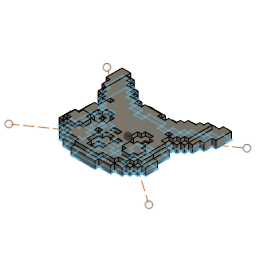
pikatchu v1 (Autodesk Fusion 360 design; units mm, degrees)
Autodesk Fusion 360 part; units mm, degrees
note: some values were not read from the file. Chosen so that the rebuilt part matches the saved one: which bodies a step acts on.
sketch "pikatchu" plane through (0, 0, 0) normal (0, 1, 0) x (1, 0, 0)
  line L0 (5, -3.5) -> (-5, 3.5) construction
  line L1 (-5, -3.5) -> (5, 3.5) construction
  line L2 (-3.9, 3.5) -> (-3.3, 3.5)
  line L3 (-3.3, 3.5) -> (-3.3, 3.2)
  line L4 (-3.3, 3.2) -> (-2.75, 3.2)
  line L5 (-2.75, 3.2) -> (-2.75, 2.9237)
  line L6 (-2.75, 2.9237) -> (-2.4765, 2.9237)
  line L7 (-2.4765, 2.9237) -> (-2.4765, 2.65)
  line L8 (-2.4765, 2.65) -> (-1.92, 2.65)
  line L9 (-1.92, 2.65) -> (-1.92, 2.365)
  line L10 (-1.92, 2.365) -> (-1.65, 2.365)
  line L11 (-1.65, 2.365) -> (-1.65, 2.1)
  line L12 (-1.65, 2.1) -> (-1.1, 2.1)
  line L13 (-1.1, 2.1) -> (-1.1, 1.8)
  line L14 (-1.1, 1.8) -> (-0.5805, 1.8)
  line L15 (-0.5805, 1.8) -> (-0.5805, 2.1)
  line L16 (-0.5805, 2.1) -> (0.5819, 2.1)
  line L17 (0.5819, 2.1) -> (0.5819, 1.8)
  line L18 (0.5819, 1.8) -> (1.1, 1.8)
  line L19 (1.1, 1.8) -> (1.1, 2.1)
  line L20 (1.1, 2.1) -> (1.65, 2.1)
  line L21 (1.65, 2.1) -> (1.65, 2.3687)
  line L22 (1.65, 2.3687) -> (1.9285, 2.3687)
  line L23 (1.9285, 2.3687) -> (1.9285, 2.65)
  line L24 (1.9285, 2.65) -> (2.4811, 2.65)
  line L25 (2.4811, 2.65) -> (2.4811, 2.9274)
  line L26 (2.4811, 2.9274) -> (2.7659, 2.9274)
  line L27 (2.7659, 2.9274) -> (2.7659, 3.2)
  line L28 (2.7659, 3.2) -> (3.3216, 3.2)
  line L29 (3.3216, 3.2) -> (3.3216, 3.4831)
  line L30 (3.3216, 3.4831) -> (3.9144, 3.4831)
  line L31 (3.9144, 3.4831) -> (3.9144, 2.3719)
  line L32 (3.9144, 2.3719) -> (3.6327, 2.3719)
  line L33 (3.6327, 2.3719) -> (3.6327, 1.8)
  line L34 (3.6327, 1.8) -> (3.3481, 1.8)
  line L35 (3.3481, 1.8) -> (3.3481, 1.2593)
  line L36 (3.3481, 1.2593) -> (3.0744, 1.2593)
  line L37 (3.0744, 1.2593) -> (3.0744, 0.9693)
  line L38 (3.0744, 0.9693) -> (2.8, 0.9693)
  line L39 (2.8, 0.9693) -> (2.8, 0.7)
  line L40 (2.8, 0.7) -> (2.523, 0.7)
  line L41 (2.523, 0.7) -> (2.523, 0.15)
  line L42 (2.523, 0.15) -> (2.8, 0.15)
  line L43 (2.8, 0.15) -> (2.8, -0.97)
  line L44 (2.8, -0.97) -> (3.08, -0.97)
  line L45 (3.08, -0.97) -> (3.08, -1.81)
  line L46 (3.08, -1.81) -> (2.8, -1.81)
  line L47 (2.8, -1.81) -> (2.8, -2.1)
  line L48 (2.8, -2.1) -> (2.52, -2.1)
  line L49 (2.52, -2.1) -> (2.52, -2.37)
  line L50 (2.52, -2.37) -> (2.24, -2.37)
  line L51 (2.24, -2.37) -> (2.24, -2.65)
  line L52 (2.24, -2.65) -> (1.69, -2.65)
  line L53 (1.69, -2.65) -> (1.69, -2.9293)
  line L54 (1.69, -2.9293) -> (0.85, -2.9293)
  line L55 (0.85, -2.9293) -> (0.85, -3.2)
  line L56 (0.85, -3.2) -> (-0.8573, -3.2)
  line L57 (-0.8573, -3.2) -> (-0.8573, -2.9293)
  line L58 (-0.8573, -2.9293) -> (-1.7, -2.9293)
  line L59 (-1.7, -2.9293) -> (-1.7, -2.65)
  line L60 (-1.7, -2.65) -> (-2.2349, -2.65)
  line L61 (-2.2349, -2.65) -> (-2.2349, -2.3726)
  line L62 (-2.2349, -2.3726) -> (-2.5262, -2.3726)
  line L63 (-2.5262, -2.3726) -> (-2.5262, -2.1)
  line L64 (-2.5262, -2.1) -> (-2.8043, -2.1)
  line L65 (-2.8043, -2.1) -> (-2.8043, -1.82)
  line L66 (-2.8043, -1.82) -> (-3.09, -1.82)
  line L67 (-3.09, -1.82) -> (-3.09, -0.9667)
  line L68 (-3.09, -0.9667) -> (-2.8043, -0.9667)
  line L69 (-2.8043, -0.9667) -> (-2.8043, 0.1465)
  line L70 (-2.8043, 0.1465) -> (-2.5283, 0.1465)
  line L71 (-2.5283, 0.1465) -> (-2.5283, 0.7)
  line L72 (-2.5283, 0.7) -> (-2.8, 0.7)
  line L73 (-2.8, 0.7) -> (-2.8, 0.966)
  line L74 (-2.8, 0.966) -> (-3.09, 0.966)
  line L75 (-3.09, 0.966) -> (-3.09, 1.24)
  line L76 (-3.09, 1.24) -> (-3.37, 1.24)
  line L77 (-3.37, 1.24) -> (-3.37, 1.8)
  line L78 (-3.37, 1.8) -> (-3.65, 1.8)
  line L79 (-3.65, 1.8) -> (-3.65, 2.36)
  line L80 (-3.65, 2.36) -> (-3.92, 2.36)
  line L81 (-3.92, 2.36) -> (-3.92, 3.5)
  line L82 (-3.92, 3.5) -> (-3.9, 3.5)
  line L83 (-2.75, 2.9237) -> (-3.05, 2.9237)
  line L84 (-3.05, 2.9237) -> (-3.05, 1.24)
  line L85 (-3.05, 1.24) -> (-2.8, 1.24)
  line L86 (-2.8, 1.24) -> (-2.8, 0.966)
  line L87 (-2.5283, 0.966) -> (-2.5283, 0.7)
  line L88 (-2.8, 0.966) -> (-2.5283, 0.966)
  line L89 (-2.5283, 0.7) -> (-2.2385, 0.7)
  line L90 (-2.2385, 0.7) -> (-2.2385, 0.9761)
  line L91 (-2.2385, 0.9761) -> (-1.95, 0.9761)
  line L92 (-1.95, 0.9761) -> (-1.95, 0.7)
  line L93 (-1.95, 0.7) -> (-2.2385, 0.7)
  line L94 (-2.2385, 0.1465) -> (-2.5283, 0.1465)
  line L95 (-2.2385, 0.7) -> (-2.2385, 0.1465)
  line L96 (-2.5283, 0.1465) -> (-2.5283, -0.9667)
  line L97 (-2.5283, -0.9667) -> (-2.8043, -0.9667)
  line L98 (-2.8043, -0.9667) -> (-2.8043, -1.82)
  line L99 (-2.8043, -1.82) -> (-2.5262, -1.82)
  line L100 (-2.5262, -1.82) -> (-2.5262, -1.2565)
  line L101 (-2.5262, -1.2565) -> (-2.2296, -1.2565)
  line L102 (-2.2296, -1.2565) -> (-2.2296, -0.9685)
  line L103 (-2.2296, -0.9685) -> (-1.7, -0.9685)
  line L104 (-1.7, -0.9685) -> (-1.7, -1.2565)
  line L105 (-1.7, -1.2565) -> (-1.4, -1.2565)
  line L106 (-1.4, -1.2565) -> (-1.4, -1.8)
  line L107 (-1.4, -1.8) -> (-1.6867, -1.8)
  line L108 (-1.6867, -1.8) -> (-1.6867, -2.1)
  line L109 (-1.6867, -2.1) -> (-2.2349, -2.1)
  line L110 (-2.2349, -2.1) -> (-2.2349, -1.82)
  line L111 (-2.2349, -1.82) -> (-2.5262, -1.82)
  line L112 (-2.5262, -1.82) -> (-2.5262, -2.1)
  line L113 (-2.5262, -2.1) -> (-2.2349, -2.1)
  line L114 (-2.2349, -2.1) -> (-2.2349, -2.3726)
  line L115 (-2.2349, -2.3726) -> (-1.7, -2.3726)
  line L116 (-1.7, -2.3726) -> (-1.7, -2.65)
  line L117 (-1.7, -2.65) -> (-0.8573, -2.65)
  line L118 (-0.8573, -2.65) -> (-0.8573, -2.9293)
  line L119 (-0.8573, -2.9293) -> (0.85, -2.9293)
  line L120 (0.85, -2.9293) -> (0.85, -2.65)
  line L121 (0.85, -2.65) -> (1.69, -2.65)
  line L122 (1.69, -2.65) -> (1.69, -2.37)
  line L123 (1.69, -2.37) -> (2.24, -2.37)
  line L124 (2.24, -2.37) -> (2.24, -2.1)
  line L125 (2.24, -2.1) -> (2.52, -2.1)
  line L126 (2.52, -2.1) -> (2.52, -1.81)
  line L127 (2.52, -1.81) -> (2.8, -1.81)
  line L128 (2.8, -0.97) -> (2.8, -1.81)
  line L129 (2.8, -0.97) -> (2.523, -0.97)
  line L130 (2.523, -0.97) -> (2.523, 0.15)
  line L131 (2.523, 0.15) -> (2.2342, 0.15)
  line L132 (2.2342, 0.15) -> (2.2342, 0.7)
  line L133 (2.2342, 0.7) -> (2.523, 0.7)
  line L134 (2.523, 0.7) -> (2.523, 0.9693)
  line L135 (2.523, 0.9693) -> (2.8, 0.9693)
  line L136 (2.2342, 0.7) -> (1.95, 0.7)
  line L137 (1.95, 0.7) -> (1.95, 0.9755)
  line L138 (1.95, 0.9755) -> (2.2342, 0.9755)
  line L139 (2.2342, 0.9755) -> (2.2342, 0.7)
  line L140 (2.8, 0.9693) -> (2.8, 1.2593)
  line L141 (2.8, 1.2593) -> (3.0744, 1.2593)
  line L142 (3.0744, 1.2593) -> (3.0744, 2.9274)
  line L143 (3.0744, 2.9274) -> (2.7659, 2.9274)
  line L144 (2.7659, 2.9274) -> (2.7659, 2.65)
  line L145 (2.7659, 2.65) -> (2.4811, 2.65)
  line L146 (2.4811, 2.65) -> (2.4811, 2.3687)
  line L147 (2.4811, 2.3687) -> (1.9285, 2.3687)
  line L148 (1.9285, 2.3687) -> (1.9285, 2.1)
  line L149 (1.9285, 2.1) -> (1.65, 2.1)
  line L150 (1.65, 2.1) -> (1.65, 1.8)
  line L151 (1.65, 1.8) -> (1.1, 1.8)
  line L152 (1.1, 1.8) -> (1.1, 1.5472)
  line L153 (1.1, 1.5472) -> (0.5819, 1.5472)
  line L154 (0.5819, 1.5472) -> (0.5819, 1.8)
  line L155 (0.5819, 1.8) -> (-0.5805, 1.8)
  line L156 (-0.5805, 1.8) -> (-0.5805, 1.55)
  line L157 (-0.5805, 1.55) -> (-1.1, 1.55)
  line L158 (-1.1, 1.55) -> (-1.1, 1.8)
  line L159 (-1.65, 2.1) -> (-1.65, 1.8)
  line L160 (-1.65, 1.8) -> (-1.1, 1.8)
  line L161 (-1.92, 2.365) -> (-1.92, 2.1)
  line L162 (-1.92, 2.1) -> (-1.65, 2.1)
  line L163 (-1.92, 2.365) -> (-2.4765, 2.365)
  line L164 (-2.4765, 2.365) -> (-2.4765, 2.65)
  line L165 (-2.75, 2.9237) -> (-2.75, 2.65)
  line L166 (-2.75, 2.65) -> (-2.4765, 2.65)
  line L167 (0.27, -2.35) -> (-0.27, -2.35)
  line L168 (-0.27, -2.35) -> (-0.27, -1.82)
  line L169 (-0.27, -1.82) -> (0.27, -1.82)
  line L170 (0.27, -1.82) -> (0.27, -2.35)
  line L171 (-0.27, -2.35) -> (-0.27, -2.65)
  line L172 (-0.27, -2.65) -> (0.27, -2.65)
  line L173 (0.27, -2.65) -> (0.27, -2.35)
  line L174 (0.27, -2.35) -> (0.5454, -2.35)
  line L175 (0.5454, -2.35) -> (0.5454, -1.5281)
  line L176 (0.5454, -1.5281) -> (0.8298, -1.5281)
  line L177 (0.8298, -1.5281) -> (0.8298, -1.2462)
  line L178 (0.8298, -1.2462) -> (0.5454, -1.2462)
  line L179 (0.5454, -1.2462) -> (0.5454, -1.5281)
  line L180 (0.2686, -1.5281) -> (0.2686, -1.2462)
  line L181 (0.2686, -1.2462) -> (-0.2864, -1.2462)
  line L182 (-0.2864, -1.2462) -> (-0.2864, -1.5281)
  line L183 (-0.2864, -1.5281) -> (-0.56, -1.5281)
  line L184 (-0.56, -1.5281) -> (-0.56, -1.2462)
  line L185 (-0.56, -1.2462) -> (-0.84, -1.2462)
  line L186 (-0.84, -1.2462) -> (-0.84, -1.5281)
  line L187 (-0.84, -1.5281) -> (-0.56, -1.5281)
  line L188 (-0.56, -1.5281) -> (-0.56, -2.35)
  line L189 (-0.56, -2.35) -> (-0.27, -2.35)
  line L190 (0.2686, -1.5281) -> (0.5454, -1.5281)
  line L191 (0.2673, -0.6984) -> (0.2673, -0.9849)
  line L192 (0.2673, -0.9849) -> (-0.2867, -0.9849)
  line L193 (-0.2867, -0.9849) -> (-0.2867, -0.6984)
  line L194 (-0.2867, -0.6984) -> (0.2673, -0.6984)
  line L195 (1.4, -1.2567) -> (1.4, -1.8)
  line L196 (1.4, -1.8) -> (1.6685, -1.8)
  line L197 (1.6685, -1.8) -> (1.6685, -2.1)
  line L198 (1.6685, -2.1) -> (2.24, -2.1)
  line L199 (2.24, -2.1) -> (2.24, -1.81)
  line L200 (2.24, -1.81) -> (2.52, -1.81)
  line L201 (2.52, -1.81) -> (2.52, -1.26)
  line L202 (2.52, -1.26) -> (2.22, -1.26)
  line L203 (2.22, -1.26) -> (2.22, -0.98)
  line L204 (2.22, -0.98) -> (1.66, -0.98)
  line L205 (1.66, -0.98) -> (1.66, -1.2567)
  line L206 (1.66, -1.2567) -> (1.4, -1.2567)
  line L207 (-1.7, -0.9685) -> (-1.1247, -0.9685)
  line L208 (-1.1247, -0.9685) -> (-1.1247, -0.69)
  line L209 (-1.1247, -0.69) -> (-0.84, -0.69)
  line L210 (-0.84, -0.69) -> (-0.84, -0.14)
  line L211 (-0.84, -0.14) -> (-1.1247, -0.14)
  line L212 (-1.1247, -0.14) -> (-1.1247, 0.14)
  line L213 (-1.1247, 0.14) -> (-1.68, 0.14)
  line L214 (-1.68, 0.14) -> (-1.68, -0.14)
  line L215 (-1.68, -0.14) -> (-1.96, -0.14)
  line L216 (-1.96, -0.14) -> (-1.96, -0.69)
  line L217 (-1.96, -0.69) -> (-1.7, -0.69)
  line L218 (-1.7, -0.69) -> (-1.7, -0.9685)
  line L219 (-1.68, -0.14) -> (-1.4, -0.14)
  line L220 (-1.4, -0.14) -> (-1.4, -0.4152)
  line L221 (-1.4, -0.4152) -> (-1.68, -0.4152)
  line L222 (-1.68, -0.4152) -> (-1.68, -0.14)
  line L223 (1.66, -0.98) -> (1.66, -0.7)
  line L224 (1.66, -0.7) -> (1.94, -0.7)
  line L225 (1.94, -0.7) -> (1.94, -0.14)
  line L226 (1.94, -0.14) -> (1.67, -0.14)
  line L227 (1.67, -0.14) -> (1.67, 0.14)
  line L228 (1.67, 0.14) -> (1.1, 0.14)
  line L229 (1.1, 0.14) -> (1.1, -0.14)
  line L230 (1.1, -0.14) -> (0.83, -0.14)
  line L231 (0.83, -0.14) -> (0.83, -0.7)
  line L232 (0.83, -0.7) -> (1.1, -0.7)
  line L233 (1.1, -0.7) -> (1.1, -0.98)
  line L234 (1.1, -0.98) -> (1.66, -0.98)
  line L235 (1.67, -0.14) -> (1.4, -0.14)
  line L236 (1.4, -0.14) -> (1.4, -0.41)
  line L237 (1.4, -0.41) -> (1.67, -0.41)
  line L238 (1.67, -0.41) -> (1.67, -0.14)
  dimension "d1" = 7
  dimension "d2" = 10
  dimension "d13" = 0.54
  constraint coincident L0 origin
  constraint coincident L1 origin
  constraint horizontal L2
  constraint perpendicular L2 L3
  constraint perpendicular L3 L4
  constraint perpendicular L4 L5
  constraint perpendicular L5 L6
  constraint perpendicular L6 L7
  constraint perpendicular L5 L8
  constraint perpendicular L8 L9
  constraint perpendicular L9 L10
  constraint perpendicular L10 L11
  constraint perpendicular L11 L12
  constraint perpendicular L10 L13
  constraint perpendicular L13 L14
  constraint perpendicular L10 L15
  constraint perpendicular L15 L16
  constraint perpendicular L16 L17
  constraint perpendicular L17 L18
  constraint perpendicular L18 L19
  constraint perpendicular L19 L20
  constraint perpendicular L18 L21
  constraint perpendicular L19 L22
  constraint perpendicular L18 L23
  constraint perpendicular L19 L24
  constraint perpendicular L18 L25
  constraint perpendicular L25 L26
  constraint perpendicular L26 L27
  constraint perpendicular L27 L28
  constraint perpendicular L26 L29
  constraint perpendicular L27 L30
  constraint perpendicular L26 L31
  constraint perpendicular L31 L32
  constraint perpendicular L26 L33
  constraint perpendicular L33 L34
  constraint perpendicular L34 L35
  constraint perpendicular L35 L36
  constraint perpendicular L36 L37
  constraint perpendicular L37 L38
  constraint perpendicular L38 L39
  constraint perpendicular L39 L40
  constraint perpendicular L38 L41
  constraint perpendicular L39 L42
  constraint perpendicular L42 L43
  constraint perpendicular L43 L44
  constraint perpendicular L42 L45
  constraint perpendicular L45 L46
  constraint perpendicular L46 L47
  constraint perpendicular L47 L48
  constraint perpendicular L46 L49
  constraint perpendicular L49 L50
  constraint perpendicular L50 L51
  constraint perpendicular L49 L52
  constraint perpendicular L52 L53
  constraint perpendicular L49 L54
  constraint perpendicular L54 L55
  constraint perpendicular L55 L56
  constraint perpendicular L56 L57
  constraint perpendicular L55 L58
  constraint perpendicular L58 L59
  constraint perpendicular L59 L60
  constraint perpendicular L60 L61
  constraint perpendicular L59 L62
  constraint perpendicular L62 L63
  constraint perpendicular L63 L64
  constraint perpendicular L64 L65
  constraint perpendicular L63 L66
  constraint perpendicular L64 L67
  constraint perpendicular L67 L68
  constraint perpendicular L68 L69
  constraint perpendicular L69 L70
  constraint perpendicular L70 L71
  constraint perpendicular L71 L72
  constraint perpendicular L70 L73
  constraint perpendicular L73 L74
  constraint perpendicular L74 L75
  constraint perpendicular L73 L76
  constraint perpendicular L74 L77
  constraint perpendicular L73 L78
  constraint perpendicular L78 L79
  constraint perpendicular L73 L80
  constraint perpendicular L80 L81
  constraint perpendicular L81 L82
  constraint perpendicular L5 L83
  constraint perpendicular L83 L84
  constraint perpendicular L84 L85
  constraint parallel L74 L88
  constraint perpendicular L87 L88
  constraint perpendicular L87 L89
  constraint perpendicular L89 L90
  constraint perpendicular L90 L91
  constraint perpendicular L91 L92
  constraint perpendicular L90 L93
  constraint parallel L92 L95
  constraint perpendicular L94 L95
  constraint perpendicular L94 L96
  constraint perpendicular L96 L97
  constraint perpendicular L66 L98
  constraint perpendicular L98 L99
  constraint perpendicular L66 L100
  constraint perpendicular L100 L101
  constraint perpendicular L101 L102
  constraint perpendicular L102 L103
  constraint perpendicular L101 L104
  constraint perpendicular L104 L105
  constraint perpendicular L105 L106
  constraint perpendicular L106 L107
  constraint perpendicular L106 L109
  constraint perpendicular L109 L110
  constraint perpendicular L110 L111
  constraint perpendicular L107 L108
  constraint perpendicular L64 L112
  constraint perpendicular L62 L114
  constraint perpendicular L61 L115
  constraint perpendicular L115 L116
  constraint perpendicular L59 L117
  constraint perpendicular L117 L118
  constraint perpendicular L55 L119
  constraint perpendicular L54 L120
  constraint perpendicular L120 L121
  constraint perpendicular L121 L122
  constraint perpendicular L122 L123
  constraint perpendicular L50 L124
  constraint perpendicular L124 L125
  constraint perpendicular L48 L126
  constraint perpendicular L126 L127
  constraint perpendicular L44 L128
  constraint perpendicular L128 L129
  constraint perpendicular L129 L130
  constraint perpendicular L130 L131
  constraint perpendicular L131 L132
  constraint perpendicular L41 L133
  constraint perpendicular L133 L134
  constraint perpendicular L134 L135
  constraint perpendicular L132 L136
  constraint perpendicular L136 L137
  constraint perpendicular L132 L138
  constraint perpendicular L133 L139
  constraint perpendicular L38 L140
  constraint perpendicular L140 L141
  constraint perpendicular L36 L142
  constraint perpendicular L142 L143
  constraint perpendicular L143 L144
  constraint perpendicular L27 L145
  constraint perpendicular L145 L146
  constraint perpendicular L146 L147
  constraint perpendicular L22 L148
  constraint perpendicular L149 L150
  constraint parallel L151 L153
  constraint perpendicular L148 L149
  constraint perpendicular L150 L151
  constraint perpendicular L152 L153
  constraint perpendicular L18 L154
  constraint perpendicular L15 L155
  constraint perpendicular L14 L156
  constraint perpendicular L15 L157
  constraint perpendicular L14 L158
  constraint perpendicular L12 L159
  constraint perpendicular L158 L160
  constraint perpendicular L10 L161
  constraint perpendicular L161 L163
  constraint perpendicular L163 L164
  constraint perpendicular L164 L166
  constraint perpendicular L165 L166
  constraint horizontal L167
  constraint perpendicular L167 L168
  constraint perpendicular L168 L169
  constraint perpendicular L167 L170
  constraint perpendicular L167 L171
  constraint perpendicular L171 L172
  constraint perpendicular L172 L173
  constraint perpendicular L173 L174
  constraint perpendicular L174 L175
  constraint perpendicular L173 L176
  constraint perpendicular L176 L177
  constraint perpendicular L173 L178
  constraint perpendicular L178 L179
  constraint perpendicular L178 L180
  constraint perpendicular L180 L181
  constraint perpendicular L178 L182
  constraint perpendicular L180 L183
  constraint perpendicular L183 L184
  constraint perpendicular L184 L185
  constraint perpendicular L185 L186
  constraint perpendicular L184 L187
  constraint perpendicular L187 L188
  constraint perpendicular L188 L189
  constraint perpendicular L179 L190
  constraint vertical L191
  constraint perpendicular L191 L192
  constraint perpendicular L192 L193
  constraint perpendicular L191 L194
  constraint perpendicular L194 L195
  constraint perpendicular L195 L196
  constraint perpendicular L194 L197
  constraint perpendicular L197 L198
  constraint perpendicular L125 L199
  constraint perpendicular L199 L200
  constraint perpendicular L127 L201
  constraint perpendicular L126 L202
  constraint perpendicular L126 L204
  constraint perpendicular L202 L203
  constraint perpendicular L204 L205
  constraint perpendicular L205 L206
  constraint perpendicular L104 L207
  constraint perpendicular L207 L208
  constraint perpendicular L208 L209
  constraint perpendicular L207 L210
  constraint perpendicular L210 L211
  constraint perpendicular L211 L212
  constraint perpendicular L212 L213
  constraint perpendicular L211 L214
  constraint perpendicular L214 L215
  constraint perpendicular L211 L216
  constraint perpendicular L214 L217
  constraint perpendicular L217 L218
  constraint perpendicular L214 L219
  constraint perpendicular L219 L220
  constraint perpendicular L214 L221
  constraint perpendicular L215 L222
  constraint perpendicular L204 L223
  constraint perpendicular L205 L224
  constraint perpendicular L204 L225
  constraint perpendicular L205 L226
  constraint perpendicular L226 L227
  constraint perpendicular L205 L228
  constraint perpendicular L226 L229
  constraint perpendicular L205 L230
  constraint perpendicular L226 L231
  constraint perpendicular L231 L232
  constraint perpendicular L226 L233
  constraint perpendicular L233 L234
  constraint perpendicular L227 L235
  constraint perpendicular L226 L236
  constraint perpendicular L227 L237
  constraint perpendicular L235 L238
  measures "d1" distance of L1.start L0.end
  measures "d2" distance of L0.end L1.end
  measures "d13" distance of L168 L170
extrude "Extrude1" add sketch "pikatchu" along normal blind 0.75 contours L83 L84 L85 L86 L87 L88 L89 L94 L95 L96 L97 L98 L99 L100 L101 L102 L103 L104 L105 L106 L107 L108 L109 L114 L115 L116 L117 L118 L119 L120 L121 L122 L123 L124 L127 L128 L129 L130 L131 L132 L133 L134 L135 L140 L141 L142 L143 L144 L145 L146 L147 L148 L149 L150 L151 L152 L153 L154 L155 L156 L157 L158 L159 L160 L161 L162 L163 L164 L165 L166 L195 L196 L197 L198 L201 L202 L203 L204 L205 L206 makes body 1
extrude "Extrude2" add sketch "pikatchu" along normal blind 0.5 separate body contours L2 L3 L4 L5 L74 L75 L76 L77 L78 L79 L80 L81 L82 L83 L84 L85 L86 | L90 L91 L92 L93 | L207 L208 L209 L210 L211 L212 L213 L214 L215 L216 L217 L218 | L223 L224 L225 L226 L227 L228 L229 L230 L231 L232 L233 L234 | L136 L137 L138 L139 | L6 L7 L165 L166 | L8 L9 L163 L164 | L10 L11 L161 L162 | L72 L73 L87 L88 | L12 L13 L159 L160 | L71 L89 L94 L95 | L69 L70 L96 L97 | L14 L156 L157 L158 | L15 L16 L17 L155 | L66 L67 L68 L98 | L18 L152 L153 L154 | L64 L65 L99 L112 | L19 L20 L150 L151 | L62 L63 L113 L114 | L21 L22 L148 L149 | L60 L61 L115 L116 | L23 L24 L146 L147 | L58 L59 L117 L118 | L25 L26 L144 L145 | L55 L56 L57 L119 | L27 L28 L29 L30 L31 L32 L33 L34 L35 L36 L142 L143 | L53 L54 L120 L121 | L37 L38 L140 L141 | L51 L52 L122 L123 | L39 L40 L134 L135 | L49 L50 L124 L125 | L41 L131 L132 L133 | L47 L48 L126 L127 | L42 L43 L129 L130 | L44 L45 L46 L128 | L167 L171 L172 L173 | L184 L185 L186 L187 | L176 L177 L178 L179 | L168 L169 L170 L174 L175 L180 L181 L182 L183 L188 L189 L190 | L191 L192 L193 L194 makes body 6 at (-3.7133, 0, -3.02) makes body 6 at (-2.75, 0.1667, -2.8325) makes body 6 at (-2.7094, 0.1667, -0.966) makes body 6 at (-2.291, 0.1667, -2.65) makes body 6 at (-2.5283, 0.1667, -0.331) makes body 6 at (-2.1423, 0.1667, -0.9761) makes body 6 at (-2.5283, 0.1667, 0.2246) makes body 6 at (-1.83, 0.1667, -2.1) makes body 6 at (-2.8043, 0.1667, 1.2511) makes body 6 at (-1.4667, 0.1667, -2.1) makes body 6 at (-2.8043, 0.1667, 2.0067) makes body 6 at (-0.9268, 0.1667, -1.8) makes body 6 at (-2.4291, 0.1667, 2.1) makes body 6 at (0.1944, 0.1667, -1.8) makes body 6 at (0.7546, 0.1667, -1.8) makes body 6 at (-2.0566, 0.1667, 2.3726) makes body 6 at (1.2833, 0.1667, -2.1) makes body 6 at (-1.4191, 0.1667, 2.65) makes body 6 at (1.8357, 0.1667, -2.1) makes body 6 at (-0.2882, 0.1667, 2.9293) makes body 6 at (2.2969, 0.1667, -2.3687) makes body 6 at (1.13, 0.1667, 2.65) makes body 6 at (2.671, 0.1667, -2.65) makes body 6 at (2.0567, 0.1667, 2.65) makes body 6 at (3.7168, 0, -3.0183) makes body 6 at (2.4267, 0.1667, 2.37) makes body 6 at (3.0744, 0.1667, -1.1626) makes body 6 at (2.52, 0.1667, 2.0033) makes body 6 at (2.6153, 0.1667, -0.9693) makes body 6 at (2.8, 0.1667, 1.25) makes body 6 at (2.8, 0.1667, 0.2233) makes body 6 at (2.523, 0.1667, -0.5167) makes body 6 at (2.1395, 0.1667, -0.7) makes body 4 at (-0.4633, 0, 1.8994) makes body 4 at (-0.09, 0.1667, 2.65) makes body 4 at (0.735, 0.1667, 1.2462) makes body 4 at (-0.56, 0.1667, 1.4341) makes body 3 at (-1.4016, 0, -0.0467) makes body 5 at (1.2, 0, 0.4167) makes body 2 at (0.0827, 0.1667, 0.9849)
extrude "Extrude3" add sketch "pikatchu" along normal blind 0.75 separate body contours L110 L111 L112 L113 | L125 L126 L199 L200 makes body 7 at (-2.4291, 0.25, 2.1) makes body 8 at (2.52, 0.25, 2.0033)
extrude "Extrude4" add sketch "pikatchu" along normal blind 1 contours L100 L101 L102 L103 L104 L105 L106 L107 L108 L109 L110 L111 | L195 L196 L197 L198 L199 L200 L201 L202 L203 L204 L205 L206 bodies 7 3 5 6 1 8
extrude "Extrude5" add sketch "pikatchu" along normal blind 0.4 separate body contours L219 L220 L221 L222 | L235 L236 L237 L238 makes body 9 at (-1.5867, 0.1333, 0.14) makes body 10 at (1.49, 0.1333, 0.41)
named bodies: "yellow"
